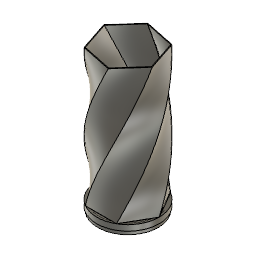
lamp hull (Autodesk Fusion 360 design; units mm, degrees)
part number: 2026-05-21-10-49-18-693
Autodesk Fusion 360 part; units mm, degrees
sketch "Sketch1" plane through (0, 0, 0) normal (0, 0, 1) x (1, 0, 0)
  circle A0 centre (0, 0) radius 38.7995
  circle A1 centre (0, 0) radius 36.9995
  dimension "d1" = 77.599
  dimension "d2" = 73.999
  constraint coincident A0.centre A1.centre
  measures "d1" diameter of A0
  measures "d2" diameter of A1
extrude "Extrude1" add sketch "Sketch1" along normal blind 4.8 from surface at 17.9
sketch "Sketch2" plane through (0, 0, 22.7) normal (0, 0, 1) x (-1, 0, 0)
  circle A0 centre (0, 0) radius 36.9995
  circle A1 centre (0, 0) radius 38.7995
  circle A2 centre (0, 0) radius 40
  dimension "d6" = 80
  constraint concentric A0 A2
  measures "d6" diameter of A2
extrude "Extrude2" add sketch "Sketch2" along normal blind 7.3 contours A1 | A2
sketch "Sketch3" plane through (0, 0, 30) normal (0, 0, 1) x (-1, 0, 0)
  circle A0 centre (0, 0) radius 36.9995
  circle A1 centre (0, 0) radius 40
  line L0 (-40, 0) -> (-20, -34.641)
  line L1 (-20, -34.641) -> (20, -34.641)
  line L2 (20, -34.641) -> (40, 0)
  line L3 (40, 0) -> (20, 34.641)
  line L4 (20, 34.641) -> (-20, 34.641)
  line L5 (-20, 34.641) -> (-40, 0)
  line L6 (38.8453, 0) -> (19.4226, 33.641)
  line L7 (19.4226, 33.641) -> (-19.4226, 33.641)
  line L8 (-19.4226, 33.641) -> (-38.8453, 0)
  line L9 (-38.8453, 0) -> (-19.4226, -33.641)
  line L10 (-19.4226, -33.641) -> (19.4226, -33.641)
  line L11 (19.4226, -33.641) -> (38.8453, 0)
  dimension "d9" = 40
  dimension "d10" = 20
  dimension "d11" = -1
  constraint coincident A0.centre A1.centre
  measures "d9" horizontal distance of L3.end L4.end
  measures "d10" horizontal distance of A0.centre L0.end
sketch "Sketch4" plane through (0, 0, 0) normal (0, 1, 0) x (1, 0, 0)
  line L0 (0, -30) -> (0, -200)
  dimension "d12" = 170
  constraint vertical L0
  measures "d12" distance of L0.start L0.end
sweep "Sweep1" add twist angle 108.3 profiles "Sketch3" path "Sketch4" along L0 section 1 contours A0 L3 L6 | A0 L2 L3 L6 L11 | A0 L2 L11 | A0 L3 L4 L6 L7 | A0 L1 L2 L10 L11 | A0 L4 L7 | A0 L1 L10 | A0 L4 L5 L7 L8 | A0 L0 L1 L9 L10 | A0 L5 L8 | A0 L0 L9 | A0 L0 L5 L8 L9
sketch "Sketch5" plane through (0, 0, 30) normal (0, 0, 1) x (-1, 0, 0)
  line L0 (-23.5007, 28.5776) -> (-20, 34.641)
  arc A0 (-20, 34.641) -> (-40, 0) centre (0, 0) ccw
  line L1 (-40, 0) -> (-36.4993, 6.0634)
  arc A1 (-23.5007, 28.5776) -> (-36.4993, 6.0634) centre (0, 0) ccw
  arc A2 (-23.5007, 28.5776) -> (-36.4993, 6.0634) centre (0, 0) ccw
  line L2 (-23.5007, 28.5776) -> (-36.4993, 6.0634)
  point P0 (-36.4993, 6.0634)
  point P1 (-23.5007, 28.5776)
extrude "Extrude3" add sketch "Sketch5" against normal blind 0.8
pattern_circular "C-Pattern1" count 6 over 360 about axis through (0, 0, 1.75) along (0, 0, 1) of "Extrude3"
